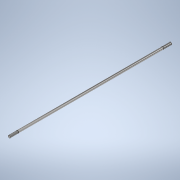
# Autodesk Inventor part: Стяжка
Saved by Autodesk Inventor 2021 (Build 250183000, 183)
## iProperties
Created: 2020-12-13
Part Number: Стяжка
Material: Сталь, высокопрочная, низколегированная
Document SubType Name: Modeling
Designer: Тимоха
Mass: 1087.57 g
Surface Area: 398.919 cm^2
Volume: 138.544 cm^3
Density: 7.85 g/cm^3
Appearance: Сталь — полированная
Author: Тимоха
Autodesk Inventor part; units mm, degrees
ref_plane "YZ Plane" through (0, 0, 0) normal (1, 0, 0) x (0, 1, 0)
ref_plane "XZ Plane" through (0, 0, 0) normal (0, 1, 0) x (-1, 0, 0)
ref_plane "XY Plane" through (0, 0, 0) normal (0, 0, 1) x (1, 0, 0)
sketch "Эскиз1" plane through (0, 0, 0) normal (0, 0, 1) x (1, 0, 0)
  circle A0 centre (0, 0) radius 7
  dimension "d0" = 14
  constraints: 1 centre point, 1 coincident
  measures "d0" diameter of A0
extrude "Выдавливание1" add sketch "Эскиз1" along normal blind 900
sketch "Эскиз2" plane through (0, 0, 0) normal (1, 0, 0) x (0, 1, 0)
  line L0 (7, 900) -> (-7, 900) projected
  line L1 (7, 0) -> (-7, 0) projected
  line L2 (0, 0) -> (0, 45)
  line L3 (0, 45) -> (7, 45)
  line L4 (7, 0) -> (7, 900) projected
  line L5 (7, 45) -> (7, 46)
  line L6 (7, 46) -> (0, 46)
  line L7 (0, 46) -> (0, 45)
  line L8 (0, 900) -> (0, 855)
  line L9 (0, 855) -> (7, 855)
  line L10 (7, 855) -> (7, 854)
  line L11 (0, -180) -> (0, 1080) projected
  line L12 (7, 854) -> (0, 854)
  line L13 (0, 855) -> (0, 854)
  line L14 (0, 46) -> (0, 45)
  line L15 (7, 46) -> (6, 46)
  line L16 (6, 46) -> (6, 45)
  line L17 (7, 855) -> (6, 855)
  line L18 (6, 854) -> (6, 855)
  dimension "d3" = 45
  dimension "d4" = 45
  dimension "d5" = 1
  constraints: 30 end point, 10 point on line, 7 perpendicular, 3 vertical, 1 collinear, 1 midpoint
  measures "d3" distance of L2.start L2.end
  measures "d4" distance of L8.start L8.end
  measures "d5" distance of L5.end L15.end
revolve "Вращение1" cut sketch "Эскиз2" angle 360 about axis through (0, 0, -10) along (0, 0, 1) contours L4 L12 L18 L9 | L4 L3 L16 L6
thread "Резьба1" size "M14x2" class "6g" standard "ANSI Metric M Profile" full length
thread "Резьба2" size "M14x2" class "6g" standard "ANSI Metric M Profile" full length
